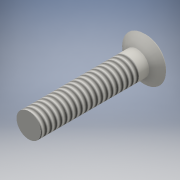
# Autodesk Inventor part: Parafuso menor Tarraxa
Saved by Autodesk Inventor 2016 (Build 200138000, 138)
## iProperties
Created: 2018-12-06
Part Number: Parafuso menor Tarraxa
Material: Generic
Document SubType Name: Sheet Metal
Designer: dqm_r
Density: 1 g/cm^3
Sheet Metal Rule: Default_mm
Appearance: Steel
Author: dqm_r
Autodesk Inventor part; units mm, degrees
ref_plane "YZ Plane" through (0, 0, 0) normal (1, 0, 0) x (0, 1, 0)
sketch "Sketch1" plane through (0, 0, 0) normal (0, 1, 0) x (-1, 0, 0)
  circle A0 centre (0, 0) radius 1.2
  dimension "d0" = 2.4
  constraints: 1 centre point, 1 coincident
  measures "d0" diameter of A0
extrude "Extrusion1" add sketch "Sketch1" along normal blind 10.6
thread "Thread1" size "M3x0.5" class "6g" standard "ANSI Metric M Profile" length 10 offset 1
ref_plane "Work Plane1" through (0, 11.3, 0) normal (0, 1, 0) x (1, 0, 0)
sketch "Sketch3" plane through (0, 11.3, 0) normal (0, 1, 0) x (1, 0, 0)
  circle A0 centre (0, 0) radius 2.15
  dimension "d6" = 4.3
  constraints: 1 centre point, 1 coincident
  measures "d6" diameter of A0
loft "Loft1" add profiles "Sketch3" section 1 edges at (1.2, 10.6, 0)
sketch "Sketch5" plane through (0, 11.3, 0) normal (0, 1, 0) x (1, 0, 0)
  circle A0 centre (0, 0) radius 2.15
  constraints: 1 centre point, 1 coincident
extrude "Extrusion2" add sketch "Sketch5" along normal blind 0.7
fillet "Fillet1" radius 2 1 edges at (-2.15, 12, 0)
ref_plane "Work Plane2" through (0, 12.1, 0) normal (0, 1, 0) x (1, 0, 0)
sketch "Sketch7" plane through (0, 12.1, 0) normal (0, 1, 0) x (1, 0, 0)
  line L0 (-1.5, -0.5) -> (-1.5, 0.5)
  line L1 (1.5, 0.5) -> (1.5, -0.5)
  line L2 (-0.5, 1.5) -> (0.5, 1.5)
  line L3 (0.5, -1.5) -> (-0.5, -1.5)
  line L4 (1.5, -0.5) -> (0.5, -0.5)
  line L5 (-0.5, -0.5) -> (-1.5, -0.5)
  line L6 (0.5, 1.5) -> (0.5, 0.5)
  line L7 (0.5, -0.5) -> (0.5, -1.5)
  line L8 (-1.5, 0.5) -> (-0.5, 0.5)
  line L9 (0.5, 0.5) -> (1.5, 0.5)
  line L10 (-0.5, -1.5) -> (-0.5, -0.5)
  line L11 (-0.5, 0.5) -> (-0.5, 1.5)
  dimension "d22" = 3
  dimension "d23" = 1
  dimension "d24" = 3
  dimension "d25" = 1
  constraints: 24 end point, 12 parallel, 4 perpendicular, 2 horizontal
  measures "d22" distance of L1.end L0.start
  measures "d23" distance of L0.start L0.end
  measures "d24" distance of L3.end L2.start
  measures "d25" distance of L2.start L2.end
extrude "Extrusion4" cut sketch "Sketch7" against normal blind 1
equation "\"BendRadius\" = Thickness"
equation "\"BendReliefWidth\" = Thickness"
equation "\"BendReliefDepth\" = 0.5 * Thickness"
equation "\"CornerReliefSize\" = 4 * Thickness"
equation "\"MinimumRemnant\" = 2 * Thickness"
equation "\"TransitionRadius\" = BendRadius"
equation "\"JacobiRadiusSize\" = BendRadius"
equation "\"GapSize\" = Thickness"
equation "\"Thickness\" = 0.5"
body "Solid1"
